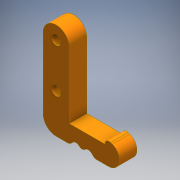
# Autodesk Inventor part: arm_lock
Saved by Autodesk Inventor 2016 (Build 200138000, 138)
## iProperties
Created: 2016-09-22
Part Number: arm_lock
Material: Nylon 6/6
Document SubType Name: Modeling
Designer: Jakub
Density: 1.13 g/cm^3
Appearance: Nylon 6
Mass: 0.72782 g
Surface Area: 6.79182 cm^2
Volume: 0.644089 cm^3
Author: Jakub
Autodesk Inventor part; units mm, degrees
ref_plane "YZ Plane" through (0, 0, 0) normal (1, 0, 0) x (0, 1, 0)
ref_plane "XZ Plane" through (0, 0, 0) normal (0, 1, 0) x (-1, 0, 0)
ref_plane "XY Plane" through (0, 0, 0) normal (0, 0, 1) x (1, 0, 0)
sketch "Sketch1" plane through (0, 0, 0) normal (0, 1, 0) x (-1, 0, 0)
  line L0 (-3, 13) -> (3, 13)
  line L1 (3, 13) -> (3, -13)
  line L2 (3, -13) -> (-3, -13)
  line L3 (-3, -13) -> (-3, 13)
  line L4 (-3, 13) -> (3, -13) construction
  line L5 (3, 13) -> (-3, -13) construction
  point P0 (0, 0)
  dimension "d0" = 6
  dimension "d1" = 26
  constraints: 12 end point, 2 midpoint, 2 parallel, 1 horizontal, 1 perpendicular
  measures "d0" distance of L1.end L2.end
  measures "d1" distance of L0.end L1.end
extrude "Extrusion1" add sketch "Sketch1" along normal blind 4
sketch "Sketch2" plane through (3, 0, -13) normal (0, 0, -1) x (-1, 0, 0)
  line L0 (0, 0) -> (6, 0) projected
  line L1 (6, 0) -> (-12, 0)
  line L2 (-12, 0) -> (-12, 4)
  line L3 (-12, 4) -> (6, 4)
  line L4 (6, 4) -> (6, 0)
  point P0 (3, 0)
  dimension "d4" = 18
  dimension "d5" = 4
  constraints: 8 end point, 2 parallel, 1 horizontal, 1 perpendicular
  measures "d4" distance of L2.end L3.end
  measures "d5" distance of L1.end L2.end
extrude "Extrusion2" add sketch "Sketch2" along normal blind 4
sketch "Sketch3" plane through (0, 4, 0) normal (0, 1, 0) x (1, 0, 0)
  line L0 (3, -13) -> (3, 13) projected
  line L1 (3, 13) -> (0, 13)
  line L2 (0, 13) -> (0, 8)
  line L3 (0, 8) -> (0, -2)
  circle A0 centre (0, 8) radius 1.1
  circle A1 centre (0, -2) radius 1.1
  point P0 (0, 0)
  dimension "d8" = 5
  dimension "d9" = 10
  dimension "d10" = 2.2
  dimension "d11" = 2.2
  constraints: 6 end point, 2 centre point, 2 coincident, 1 horizontal, 1 perpendicular, 1 point on line
  measures "d8" distance of L1.end L2.end
  measures "d9" distance of L2.end L3.end
  measures "d10" diameter of A0
  measures "d11" diameter of A1
extrude "Extrusion3" cut sketch "Sketch3" against normal up to next
sketch "Sketch4" plane through (0, 4, 0) normal (0, 1, 0) x (1, 0, 0)
  line L0 (3, 13) -> (3, -13) projected
  line L1 (-3, -13) -> (-3, 17) projected
  line L2 (3, -13) -> (-3, -13)
  line L3 (-3, -13) -> (-3, -5)
  line L4 (-3, -5) -> (3, -5)
  line L5 (3, -5) -> (3, -13)
  point P0 (0, 0)
  dimension "d14" = 8
  constraints: 8 end point, 2 parallel, 1 horizontal, 1 perpendicular, 1 point on line
  measures "d14" distance of L2.end L3.end
extrude "Extrusion4" cut sketch "Sketch4" against normal blind 4
fillet "Fillet1" radius 3 2 edges at (3, 2, 5) (-3, 2, 5)
sketch "Sketch5" plane through (0, 4, 0) normal (0, 1, 0) x (1, 0, 0)
  line L0 (15, 13) -> (11.1, 13)
  line L1 (3, 13) -> (15, 13) projected
  line L2 (11.1, 13) -> (11.1, 11.5)
  line L3 (11.1, 11.5) -> (15, 13)
  point P0 (0, 0)
  dimension "d18" = 3.9
  dimension "d19" = 1.5
  constraints: 6 end point, 1 perpendicular, 1 point on line
  measures "d18" distance of L0.start L0.end
  measures "d19" distance of L0.end L2.end
extrude "Extrusion5" add sketch "Sketch5" against normal blind 4
fillet "Fillet2" radius 1 1 edges at (11.1, 2, -11.5)
fillet "Fillet3" radius 3 1 edges at (-3, 2, -17)
sketch "Sketch6" plane through (0, 4, 0) normal (0, 1, 0) x (1, 0, 0)
  line L0 (0, 17) -> (15, 17) projected
  line L1 (3.0924, 17) -> (4.5066, 15.5858)
  line L2 (3.0924, 17) -> (5.0924, 17) construction
  line L3 (4.5066, 15.5858) -> (5.9208, 17)
  line L4 (5.9208, 17) -> (7.335, 15.5858)
  line L5 (5.9208, 17) -> (7.9208, 17) construction
  line L6 (7.335, 15.5858) -> (8.7492, 17)
  point P0 (0, 0)
  dimension "d24" = 2
  dimension "d25" = 45
  dimension "d26" = 2
  dimension "d27" = 45
  constraints: 12 end point, 3 point on line, 2 equal length, 2 horizontal, 1 perpendicular
  measures "d24" distance of L1.start L1.end
  measures "d25" angle of L1 L2
  measures "d26" distance of L3.end L4.end
  measures "d27" angle of L4 L5
extrude "Extrusion6" cut sketch "Sketch6" against normal up to next
fillet "Fillet4" radius 1 5 edges at (3.0924, 2, -17) (4.5066, 2, -15.5858) (5.9208, 2, -17) (7.335, 2, -15.5858) (8.7492, 2, -17)
fillet "Fillet5" radius 2.5 2 edges at (15, 2, -17) (15, 2, -13)
body "Solid1"
